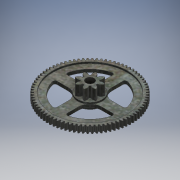
# Autodesk Inventor part: 足 初段焼結ギア　80-8
Saved by Autodesk Inventor 2016 (Build 200138000, 138)
## iProperties
Created: 2018-04-22
Part Number: 足 初段焼結ギア　80-8
Material: 鋼
Document SubType Name: Modeling
Designer: Takumi
Density: 7.85 g/cm^3
Appearance: プレート
Mass: 15.2958 g
Surface Area: 32.495 cm^2
Volume: 1.9485 cm^3
Author: Takumi
Autodesk Inventor part; units mm, degrees
(part 1 of 7)
ref_plane "YZ Plane" through (0, 0, 0) normal (1, 0, 0) x (0, 1, 0)
ref_plane "XZ Plane" through (0, 0, 0) normal (0, 1, 0) x (-1, 0, 0)
ref_plane "XY Plane" through (0, 0, 0) normal (0, 0, 1) x (1, 0, 0)
sketch "スケッチ1" plane through (0, 0, 0) normal (0, 0, 1) x (1, 0, 0)
  arc A0 (148.7771, 124.6719) -> (148.6896, 124.3741) centre (153.7892, 123.0371) ccw
  arc A1 (148.9109, 125.0429) -> (148.7771, 124.6719) centre (154.869, 122.6849) ccw
  arc A2 (149.1052, 125.4911) -> (148.9109, 125.0429) centre (155.9658, 122.2508) ccw
  arc A3 (147.2329, 124.633) -> (147.169, 124.3292) centre (152.3577, 123.3965) ccw
  arc A4 (147.3371, 125.0133) -> (147.2329, 124.633) centre (153.4618, 123.1301) ccw
  arc A5 (147.4956, 125.4754) -> (147.3371, 125.0133) centre (154.5894, 122.7834) ccw
  arc A6 (145.6964, 124.473) -> (145.6565, 124.1652) centre (150.9025, 123.6425) ccw
  arc A7 (145.7705, 124.8604) -> (145.6964, 124.473) centre (152.0241, 123.4635) ccw
  arc A8 (145.8922, 125.3335) -> (145.7705, 124.8604) centre (153.1753, 123.2064) ccw
  arc A9 (144.1772, 124.193) -> (144.1616, 123.883) centre (149.4324, 123.7735) ccw
  arc A10 (144.2207, 124.585) -> (144.1772, 124.193) centre (150.5646, 123.6831) ccw
  arc A11 (144.3049, 125.0662) -> (144.2207, 124.585) centre (151.7324, 123.517) ccw
  arc A12 (142.6846, 123.7947) -> (142.6934, 123.4844) centre (147.9566, 123.7888) ccw
  arc A13 (142.6972, 124.1889) -> (142.6846, 123.7947) centre (149.0924, 123.7875) ccw
  arc A14 (142.7435, 124.6752) -> (142.6972, 124.1889) centre (150.2696, 123.7136) ccw
  arc A15 (141.228, 123.2805) -> (141.2611, 122.9719) centre (146.4841, 123.6882) ccw
  arc A16 (141.2096, 123.6745) -> (141.228, 123.2805) centre (147.6165, 123.776) ccw
  arc A17 (141.2175, 124.1629) -> (141.2096, 123.6745) centre (148.7959, 123.7947) ccw
  arc A18 (139.8161, 122.6536) -> (139.8733, 122.3485) centre (145.024, 123.4724) ccw
  arc A19 (139.7669, 123.0449) -> (139.8161, 122.6536) centre (146.1461, 123.6488) ccw
  arc A20 (139.7365, 123.5324) -> (139.7669, 123.0449) centre (147.3204, 123.76) ccw
  arc A21 (138.4578, 121.9178) -> (138.5388, 121.6182) centre (143.5854, 123.1428) ccw
  arc A22 (138.378, 122.3041) -> (138.4578, 121.9178) centre (144.6901, 123.4067) ccw
  arc A23 (138.3095, 122.7877) -> (138.378, 122.3041) centre (145.8522, 123.6096) ccw
  arc A24 (137.1614, 121.0778) -> (137.2656, 120.7854) centre (142.1771, 122.7012) ccw
  arc A25 (137.0515, 121.4566) -> (137.1614, 121.0778) centre (143.2577, 123.051) ccw
  arc A26 (136.9453, 121.9334) -> (137.0515, 121.4566) centre (144.4002, 123.3445) ccw
  arc A27 (135.9349, 120.1386) -> (136.0617, 119.8553) centre (140.8078, 122.1506) ccw
  arc A28 (135.7957, 120.5076) -> (135.9349, 120.1386) centre (141.8576, 122.5841) ccw
  arc A29 (135.6523, 120.9746) -> (135.7957, 120.5076) centre (142.9736, 122.9663) ccw
  arc A30 (134.7859, 119.1061) -> (134.9345, 118.8336) centre (139.4859, 121.4942) ccw
  arc A31 (134.6181, 119.463) -> (134.7859, 119.1061) centre (140.4985, 122.0087) ccw
  arc A32 (134.4386, 119.9173) -> (134.6181, 119.463) centre (141.581, 122.4773) ccw
  arc A33 (133.7214, 117.9866) -> (133.891, 117.7266) centre (138.2195, 120.7361) ccw
  arc A34 (133.5261, 118.3293) -> (133.7214, 117.9866) centre (139.1886, 121.3285) ccw
  arc A35 (133.3115, 118.7681) -> (133.5261, 118.3293) centre (140.2311, 121.8806) ccw
  arc A36 (132.748, 116.7871) -> (132.9375, 116.5412) centre (137.0166, 119.881) ccw
  arc A37 (132.5265, 117.1134) -> (132.748, 116.7871) centre (137.9362, 120.5476) ccw
  arc A38 (132.2781, 117.534) -> (132.5265, 117.1134) centre (138.9321, 121.1798) ccw
  arc A39 (131.8718, 115.5148) -> (132.08, 115.2846) centre (135.8844, 118.9341) ccw
  arc A40 (131.6253, 115.8227) -> (131.8718, 115.5148) centre (136.7489, 119.6708) ccw
  arc A41 (131.3447, 116.2226) -> (131.6253, 115.8227) centre (137.6922, 120.3792) ccw
  arc A42 (131.0981, 114.1778) -> (131.3237, 113.9646) centre (134.8301, 117.9014) ccw
  arc A43 (130.8282, 114.4654) -> (131.0981, 114.1778) centre (135.6341, 118.7036) ccw
  arc A44 (130.5171, 114.842) -> (130.8282, 114.4654) centre (136.5188, 119.4838) ccw
  arc A45 (130.4316, 112.7842) -> (130.6733, 112.5893) centre (133.86, 116.7891) ccw
  arc A46 (130.14, 113.0497) -> (130.4316, 112.7842) centre (134.5986, 117.6519) ccw
  arc A47 (129.8003, 113.4007) -> (130.14, 113.0497) centre (135.4194, 118.4991) ccw
  arc A48 (129.8766, 111.3425) -> (130.1328, 111.1673) centre (132.9801, 115.6041) ccw
  arc A49 (129.5651, 111.5844) -> (129.8766, 111.3425) centre (133.6488, 116.5222) ccw
  arc A50 (129.1989, 111.9077) -> (129.5651, 111.5844) centre (134.4006, 117.4312) ccw
  arc A51 (129.4364, 109.8618) -> (129.7055, 109.7072) centre (132.196, 114.3537) ccw
  arc A52 (129.1068, 110.0785) -> (129.4364, 109.8618) centre (132.7905, 115.3215) ccw
  arc A53 (128.7164, 110.372) -> (129.1068, 110.0785) centre (133.4687, 116.2867) ccw
  arc A54 (129.1137, 108.3511) -> (129.3941, 108.2181) centre (131.5124, 113.0457) ccw
  arc A55 (128.7682, 108.5413) -> (129.1137, 108.3511) centre (132.0292, 114.0571) ccw
  arc A56 (128.3559, 108.8033) -> (128.7682, 108.5413) centre (132.6295, 115.0726) ccw
  arc A57 (128.9105, 106.8197) -> (129.2005, 106.7091) centre (130.9335, 111.6881) ccw
  arc A58 (128.5511, 106.9822) -> (128.9105, 106.8197) centre (131.3693, 112.7369) ccw
  arc A59 (128.1196, 107.2111) -> (128.5511, 106.9822) centre (131.8881, 113.7963) ccw
  arc A60 (128.8281, 105.2771) -> (129.1259, 105.1896) centre (130.4629, 110.2892) ccw
  arc A61 (128.4571, 105.4109) -> (128.8281, 105.2771) centre (130.8151, 111.369) ccw
  arc A62 (128.0089, 105.6052) -> (128.4571, 105.4109) centre (131.2492, 112.4658) ccw
  arc A63 (128.867, 103.7329) -> (129.1708, 103.669) centre (130.1035, 108.8577) ccw
  arc A64 (128.4867, 103.8371) -> (128.867, 103.7329) centre (130.3699, 109.9618) ccw
  arc A65 (128.0246, 103.9956) -> (128.4867, 103.8371) centre (130.7166, 111.0894) ccw
  arc A66 (129.027, 102.1964) -> (129.3348, 102.1565) centre (129.8575, 107.4025) ccw
  arc A67 (128.6396, 102.2705) -> (129.027, 102.1964) centre (130.0365, 108.5241) ccw
  arc A68 (128.1665, 102.3922) -> (128.6396, 102.2705) centre (130.2936, 109.6753) ccw
  arc A69 (129.307, 100.6772) -> (129.617, 100.6616) centre (129.7265, 105.9324) ccw
  arc A70 (128.915, 100.7207) -> (129.307, 100.6772) centre (129.8169, 107.0646) ccw
  arc A71 (128.4338, 100.8049) -> (128.915, 100.7207) centre (129.983, 108.2324) ccw
  arc A72 (129.7053, 99.1846) -> (130.0156, 99.1934) centre (129.7112, 104.4566) ccw
  arc A73 (129.3111, 99.1972) -> (129.7053, 99.1846) centre (129.7125, 105.5924) ccw
  arc A74 (128.8248, 99.2435) -> (129.3111, 99.1972) centre (129.7864, 106.7696) ccw
  arc A75 (130.2195, 97.728) -> (130.5281, 97.7611) centre (129.8118, 102.9841) ccw
  arc A76 (129.8255, 97.7096) -> (130.2195, 97.728) centre (129.724, 104.1165) ccw
  arc A77 (129.3371, 97.7175) -> (129.8255, 97.7096) centre (129.7053, 105.2959) ccw
  arc A78 (130.8464, 96.3161) -> (131.1515, 96.3733) centre (130.0276, 101.524) ccw
  arc A79 (130.4551, 96.2669) -> (130.8464, 96.3161) centre (129.8512, 102.6461) ccw
  arc A80 (129.9676, 96.2365) -> (130.4551, 96.2669) centre (129.74, 103.8204) ccw
  arc A81 (131.5822, 94.9578) -> (131.8818, 95.0388) centre (130.3572, 100.0854) ccw
  arc A82 (131.1959, 94.878) -> (131.5822, 94.9578) centre (130.0933, 101.1901) ccw
  arc A83 (130.7123, 94.8095) -> (131.1959, 94.878) centre (129.8904, 102.3522) ccw
  arc A84 (132.4222, 93.6614) -> (132.7146, 93.7656) centre (130.7988, 98.6771) ccw
  arc A85 (132.0434, 93.5515) -> (132.4222, 93.6614) centre (130.449, 99.7577) ccw
  arc A86 (131.5666, 93.4453) -> (132.0434, 93.5515) centre (130.1555, 100.9002) ccw
  arc A87 (133.3614, 92.4349) -> (133.6447, 92.5617) centre (131.3494, 97.3078) ccw
  arc A88 (132.9924, 92.2957) -> (133.3614, 92.4349) centre (130.9159, 98.3576) ccw
  arc A89 (132.5254, 92.1523) -> (132.9924, 92.2957) centre (130.5337, 99.4736) ccw
  arc A90 (134.3939, 91.2859) -> (134.6664, 91.4345) centre (132.0058, 95.9859) ccw
  arc A91 (134.037, 91.1181) -> (134.3939, 91.2859) centre (131.4913, 96.9985) ccw
  arc A92 (133.5827, 90.9386) -> (134.037, 91.1181) centre (131.0227, 98.081) ccw
  arc A93 (135.5134, 90.2214) -> (135.7734, 90.391) centre (132.7639, 94.7195) ccw
  arc A94 (135.1707, 90.0261) -> (135.5134, 90.2214) centre (132.1715, 95.6886) ccw
  arc A95 (134.7319, 89.8115) -> (135.1707, 90.0261) centre (131.6194, 96.7311) ccw
  arc A96 (136.7129, 89.248) -> (136.9588, 89.4375) centre (133.619, 93.5166) ccw
  arc A97 (136.3866, 89.0265) -> (136.7129, 89.248) centre (132.9524, 94.4362) ccw
  arc A98 (135.966, 88.7781) -> (136.3866, 89.0265) centre (132.3202, 95.4321) ccw
  arc A99 (137.9852, 88.3718) -> (138.2154, 88.58) centre (134.5659, 92.3844) ccw
  arc A100 (137.6773, 88.1253) -> (137.9852, 88.3718) centre (133.8292, 93.2489) ccw
  arc A101 (137.2774, 87.8447) -> (137.6773, 88.1253) centre (133.1208, 94.1922) ccw
  arc A102 (139.3222, 87.5981) -> (139.5354, 87.8237) centre (135.5986, 91.3301) ccw
  arc A103 (139.0346, 87.3282) -> (139.3222, 87.5981) centre (134.7964, 92.1341) ccw
  arc A104 (138.658, 87.0171) -> (139.0346, 87.3282) centre (134.0162, 93.0188) ccw
  arc A105 (140.7158, 86.9316) -> (140.9107, 87.1733) centre (136.7109, 90.36) ccw
  arc A106 (140.4503, 86.64) -> (140.7158, 86.9316) centre (135.8481, 91.0986) ccw
  arc A107 (140.0993, 86.3003) -> (140.4503, 86.64) centre (135.0009, 91.9194) ccw
  arc A108 (142.1575, 86.3766) -> (142.3327, 86.6328) centre (137.8959, 89.4801) ccw
  arc A109 (141.9156, 86.0651) -> (142.1575, 86.3766) centre (136.9778, 90.1488) ccw
  arc A110 (141.5923, 85.6989) -> (141.9156, 86.0651) centre (136.0688, 90.9006) ccw
  arc A111 (143.6382, 85.9364) -> (143.7928, 86.2055) centre (139.1463, 88.696) ccw
  arc A112 (143.4215, 85.6068) -> (143.6382, 85.9364) centre (138.1785, 89.2905) ccw
  arc A113 (143.128, 85.2164) -> (143.4215, 85.6068) centre (137.2133, 89.9687) ccw
  arc A114 (145.1489, 85.6137) -> (145.2819, 85.8941) centre (140.4543, 88.0124) ccw
  arc A115 (144.9587, 85.2682) -> (145.1489, 85.6137) centre (139.4429, 88.5292) ccw
  arc A116 (144.6967, 84.8559) -> (144.9587, 85.2682) centre (138.4274, 89.1295) ccw
  arc A117 (146.6803, 85.4105) -> (146.7909, 85.7005) centre (141.8119, 87.4335) ccw
  arc A118 (146.5178, 85.0511) -> (146.6803, 85.4105) centre (140.7631, 87.8693) ccw
  arc A119 (146.2889, 84.6196) -> (146.5178, 85.0511) centre (139.7037, 88.3881) ccw
  arc A120 (148.2229, 85.3281) -> (148.3104, 85.6259) centre (143.2108, 86.9629) ccw
  arc A121 (148.0891, 84.9571) -> (148.2229, 85.3281) centre (142.131, 87.3151) ccw
  arc A122 (147.8948, 84.5089) -> (148.0891, 84.9571) centre (141.0342, 87.7492) ccw
  arc A123 (149.7671, 85.367) -> (149.831, 85.6708) centre (144.6423, 86.6035) ccw
  arc A124 (149.6629, 84.9867) -> (149.7671, 85.367) centre (143.5382, 86.8699) ccw
  arc A125 (149.5044, 84.5246) -> (149.6629, 84.9867) centre (142.4106, 87.2166) ccw
  arc A126 (151.3036, 85.527) -> (151.3435, 85.8348) centre (146.0975, 86.3575) ccw
  arc A127 (151.2295, 85.1396) -> (151.3036, 85.527) centre (144.9759, 86.5365) ccw
  arc A128 (151.1078, 84.6665) -> (151.2295, 85.1396) centre (143.8247, 86.7936) ccw
  arc A129 (152.8228, 85.807) -> (152.8384, 86.117) centre (147.5676, 86.2265) ccw
  arc A130 (152.7793, 85.415) -> (152.8228, 85.807) centre (146.4354, 86.3169) ccw
  arc A131 (152.6951, 84.9338) -> (152.7793, 85.415) centre (145.2676, 86.483) ccw
  arc A132 (154.3154, 86.2053) -> (154.3066, 86.5156) centre (149.0434, 86.2112) ccw
  arc A133 (154.3028, 85.8111) -> (154.3154, 86.2053) centre (147.9076, 86.2125) ccw
  arc A134 (154.2565, 85.3248) -> (154.3028, 85.8111) centre (146.7304, 86.2864) ccw
  arc A135 (155.772, 86.7195) -> (155.7389, 87.0281) centre (150.5159, 86.3118) ccw
  arc A136 (155.7904, 86.3255) -> (155.772, 86.7195) centre (149.3835, 86.224) ccw
  arc A137 (155.7825, 85.8371) -> (155.7904, 86.3255) centre (148.2041, 86.2053) ccw
  arc A138 (157.1839, 87.3464) -> (157.1267, 87.6515) centre (151.976, 86.5276) ccw
  arc A139 (157.2331, 86.9551) -> (157.1839, 87.3464) centre (150.8539, 86.3512) ccw
  arc A140 (157.2635, 86.4676) -> (157.2331, 86.9551) centre (149.6796, 86.24) ccw
  arc A141 (158.5422, 88.0822) -> (158.4612, 88.3818) centre (153.4146, 86.8572) ccw
  arc A142 (158.622, 87.6959) -> (158.5422, 88.0822) centre (152.3099, 86.5933) ccw
  arc A143 (158.6905, 87.2123) -> (158.622, 87.6959) centre (151.1478, 86.3904) ccw
  arc A144 (159.8386, 88.9222) -> (159.7344, 89.2146) centre (154.8229, 87.2988) ccw
  arc A145 (159.9485, 88.5434) -> (159.8386, 88.9222) centre (153.7423, 86.949) ccw
  arc A146 (160.0547, 88.0666) -> (159.9485, 88.5434) centre (152.5998, 86.6555) ccw
  arc A147 (161.0651, 89.8614) -> (160.9383, 90.1447) centre (156.1922, 87.8494) ccw
  arc A148 (161.2043, 89.4924) -> (161.0651, 89.8614) centre (155.1424, 87.4159) ccw
  arc A149 (161.3477, 89.0254) -> (161.2043, 89.4924) centre (154.0264, 87.0337) ccw
  arc A150 (162.2141, 90.8939) -> (162.0655, 91.1664) centre (157.5141, 88.5058) ccw
  arc A151 (162.3819, 90.537) -> (162.2141, 90.8939) centre (156.5015, 87.9913) ccw
  arc A152 (162.5614, 90.0827) -> (162.3819, 90.537) centre (155.419, 87.5227) ccw
  arc A153 (163.2786, 92.0134) -> (163.109, 92.2734) centre (158.7805, 89.2639) ccw
  arc A154 (163.4738, 91.6707) -> (163.2786, 92.0134) centre (157.8114, 88.6715) ccw
  arc A155 (163.6885, 91.2319) -> (163.4738, 91.6707) centre (156.7689, 88.1194) ccw
  arc A156 (164.252, 93.2129) -> (164.0625, 93.4588) centre (159.9834, 90.119) ccw
  arc A157 (164.4735, 92.8866) -> (164.252, 93.2129) centre (159.0638, 89.4524) ccw
  arc A158 (164.7219, 92.466) -> (164.4735, 92.8866) centre (158.0679, 88.8202) ccw
  arc A159 (165.1282, 94.4852) -> (164.92, 94.7154) centre (161.1156, 91.0659) ccw
  arc A160 (165.3747, 94.1773) -> (165.1282, 94.4852) centre (160.2511, 90.3292) ccw
  arc A161 (165.6553, 93.7774) -> (165.3747, 94.1773) centre (159.3078, 89.6208) ccw
  arc A162 (165.9019, 95.8222) -> (165.6763, 96.0354) centre (162.1699, 92.0986) ccw
  arc A163 (166.1718, 95.5346) -> (165.9019, 95.8222) centre (161.3659, 91.2964) ccw
  arc A164 (166.4829, 95.158) -> (166.1718, 95.5346) centre (160.4812, 90.5162) ccw
  arc A165 (166.5684, 97.2158) -> (166.3267, 97.4107) centre (163.14, 93.2109) ccw
  arc A166 (166.86, 96.9503) -> (166.5684, 97.2158) centre (162.4014, 92.3481) ccw
  arc A167 (167.1997, 96.5993) -> (166.86, 96.9503) centre (161.5806, 91.5009) ccw
  arc A168 (167.1234, 98.6575) -> (166.8672, 98.8327) centre (164.0199, 94.3959) ccw
  arc A169 (167.4349, 98.4156) -> (167.1234, 98.6575) centre (163.3512, 93.4778) ccw
  arc A170 (167.8011, 98.0923) -> (167.4349, 98.4156) centre (162.5994, 92.5688) ccw
  arc A171 (167.5636, 100.1382) -> (167.2945, 100.2928) centre (164.804, 95.6463) ccw
  arc A172 (167.8932, 99.9215) -> (167.5636, 100.1382) centre (164.2095, 94.6785) ccw
  arc A173 (168.2836, 99.628) -> (167.8932, 99.9215) centre (163.5313, 93.7133) ccw
  arc A174 (167.8863, 101.6489) -> (167.6059, 101.7819) centre (165.4876, 96.9543) ccw
  arc A175 (168.2318, 101.4587) -> (167.8863, 101.6489) centre (164.9708, 95.9429) ccw
  arc A176 (168.6441, 101.1967) -> (168.2318, 101.4587) centre (164.3705, 94.9274) ccw
  arc A177 (168.0895, 103.1803) -> (167.7995, 103.2909) centre (166.0665, 98.3119) ccw
  arc A178 (168.4489, 103.0178) -> (168.0895, 103.1803) centre (165.6307, 97.2631) ccw
  arc A179 (168.8804, 102.7889) -> (168.4489, 103.0178) centre (165.1119, 96.2037) ccw
  arc A180 (168.1719, 104.7229) -> (167.8741, 104.8104) centre (166.5371, 99.7108) ccw
  arc A181 (168.5429, 104.5891) -> (168.1719, 104.7229) centre (166.1849, 98.631) ccw
  arc A182 (168.9911, 104.3948) -> (168.5429, 104.5891) centre (165.7508, 97.5342) ccw
  arc A183 (168.133, 106.2671) -> (167.8292, 106.331) centre (166.8965, 101.1423) ccw
  arc A184 (168.5133, 106.1629) -> (168.133, 106.2671) centre (166.6301, 100.0382) ccw
  arc A185 (168.9754, 106.0044) -> (168.5133, 106.1629) centre (166.2834, 98.9106) ccw
  arc A186 (167.973, 107.8036) -> (167.6652, 107.8435) centre (167.1425, 102.5975) ccw
  arc A187 (168.3604, 107.7295) -> (167.973, 107.8036) centre (166.9635, 101.4759) ccw
  arc A188 (168.8335, 107.6078) -> (168.3604, 107.7295) centre (166.7064, 100.3247) ccw
  arc A189 (167.693, 109.3228) -> (167.383, 109.3384) centre (167.2735, 104.0676) ccw
  arc A190 (168.085, 109.2793) -> (167.693, 109.3228) centre (167.1831, 102.9354) ccw
  arc A191 (168.5662, 109.1951) -> (168.085, 109.2793) centre (167.017, 101.7676) ccw
  arc A192 (167.2947, 110.8154) -> (166.9844, 110.8066) centre (167.2888, 105.5434) ccw
  arc A193 (167.6889, 110.8028) -> (167.2947, 110.8154) centre (167.2875, 104.4076) ccw
  arc A194 (168.1752, 110.7565) -> (167.6889, 110.8028) centre (167.2136, 103.2304) ccw
  arc A195 (166.7805, 112.272) -> (166.4719, 112.2389) centre (167.1882, 107.0159) ccw
  arc A196 (167.1745, 112.2904) -> (166.7805, 112.272) centre (167.276, 105.8835) ccw
  arc A197 (167.6629, 112.2825) -> (167.1745, 112.2904) centre (167.2947, 104.7041) ccw
  arc A198 (166.1536, 113.6839) -> (165.8485, 113.6267) centre (166.9724, 108.476) ccw
  arc A199 (166.5449, 113.7331) -> (166.1536, 113.6839) centre (167.1488, 107.3539) ccw
  arc A200 (167.0324, 113.7635) -> (166.5449, 113.7331) centre (167.26, 106.1796) ccw
  arc A201 (165.4178, 115.0422) -> (165.1182, 114.9612) centre (166.6428, 109.9146) ccw
  arc A202 (165.8041, 115.122) -> (165.4178, 115.0422) centre (166.9067, 108.8099) ccw
  arc A203 (166.2877, 115.1905) -> (165.8041, 115.122) centre (167.1096, 107.6478) ccw
  arc A204 (164.5778, 116.3386) -> (164.2854, 116.2344) centre (166.2012, 111.3229) ccw
  arc A205 (164.9566, 116.4485) -> (164.5778, 116.3386) centre (166.551, 110.2423) ccw
  arc A206 (165.4334, 116.5547) -> (164.9566, 116.4485) centre (166.8445, 109.0998) ccw
  arc A207 (163.6386, 117.5651) -> (163.3553, 117.4383) centre (165.6506, 112.6922) ccw
  arc A208 (164.0076, 117.7043) -> (163.6386, 117.5651) centre (166.0841, 111.6424) ccw
  arc A209 (164.4746, 117.8477) -> (164.0076, 117.7043) centre (166.4663, 110.5264) ccw
  arc A210 (162.6061, 118.7141) -> (162.3336, 118.5655) centre (164.9942, 114.0141) ccw
  arc A211 (162.963, 118.8819) -> (162.6061, 118.7141) centre (165.5087, 113.0015) ccw
  arc A212 (163.4173, 119.0614) -> (162.963, 118.8819) centre (165.9773, 111.919) ccw
  arc A213 (161.4866, 119.7786) -> (161.2266, 119.609) centre (164.2361, 115.2805) ccw
  arc A214 (161.8293, 119.9739) -> (161.4866, 119.7786) centre (164.8285, 114.3114) ccw
  arc A215 (162.2681, 120.1885) -> (161.8293, 119.9739) centre (165.3806, 113.2689) ccw
  arc A216 (160.2871, 120.752) -> (160.0412, 120.5625) centre (163.381, 116.4834) ccw
  arc A217 (160.6134, 120.9735) -> (160.2871, 120.752) centre (164.0476, 115.5638) ccw
  arc A218 (161.034, 121.2219) -> (160.6134, 120.9735) centre (164.6798, 114.5679) ccw
  arc A219 (159.0148, 121.6282) -> (158.7846, 121.42) centre (162.4341, 117.6156) ccw
  arc A220 (159.3227, 121.8747) -> (159.0148, 121.6282) centre (163.1708, 116.7511) ccw
  arc A221 (159.7226, 122.1553) -> (159.3227, 121.8747) centre (163.8792, 115.8078) ccw
  arc A222 (157.6778, 122.4019) -> (157.4646, 122.1763) centre (161.4014, 118.6699) ccw
  arc A223 (157.9654, 122.6718) -> (157.6778, 122.4019) centre (162.2036, 117.8659) ccw
  arc A224 (158.342, 122.9829) -> (157.9654, 122.6718) centre (162.9838, 116.9812) ccw
  arc A225 (156.2842, 123.0684) -> (156.0893, 122.8267) centre (160.2891, 119.64) ccw
  arc A226 (156.5497, 123.36) -> (156.2842, 123.0684) centre (161.1519, 118.9014) ccw
  arc A227 (156.9007, 123.6997) -> (156.5497, 123.36) centre (161.9991, 118.0806) ccw
  arc A228 (154.8425, 123.6234) -> (154.6673, 123.3672) centre (159.1041, 120.5199) ccw
  arc A229 (155.0844, 123.9349) -> (154.8425, 123.6234) centre (160.0222, 119.8512) ccw
  arc A230 (155.4077, 124.3011) -> (155.0844, 123.9349) centre (160.9312, 119.0994) ccw
  arc A231 (153.3618, 124.0636) -> (153.2072, 123.7945) centre (157.8537, 121.304) ccw
  arc A232 (153.5785, 124.3932) -> (153.3618, 124.0636) centre (158.8215, 120.7095) ccw
  arc A233 (153.872, 124.7836) -> (153.5785, 124.3932) centre (159.7867, 120.0313) ccw
  arc A234 (151.8511, 124.3863) -> (151.7181, 124.1059) centre (156.5457, 121.9876) ccw
  arc A235 (152.0413, 124.7318) -> (151.8511, 124.3863) centre (157.5571, 121.4708) ccw
  arc A236 (152.3033, 125.1441) -> (152.0413, 124.7318) centre (158.5726, 120.8705) ccw
  arc A237 (150.3197, 124.5895) -> (150.2091, 124.2995) centre (155.1881, 122.5665) ccw
  arc A238 (150.4822, 124.9489) -> (150.3197, 124.5895) centre (156.2369, 122.1307) ccw
  arc A239 (150.7111, 125.3804) -> (150.4822, 124.9489) centre (157.2963, 121.6119) ccw
  arc A240 (148.3104, 124.3741) -> (148.2229, 124.6719) centre (143.2108, 123.0371) ccw
  arc A241 (148.2229, 124.6719) -> (148.0891, 125.0429) centre (142.131, 122.6849) ccw
  arc A242 (148.0891, 125.0429) -> (147.8948, 125.4911) centre (141.0342, 122.2508) ccw
  arc A243 (146.7909, 124.2995) -> (146.6803, 124.5895) centre (141.8119, 122.5665) ccw
  arc A244 (146.6803, 124.5895) -> (146.5178, 124.9489) centre (140.7631, 122.1307) ccw
  arc A245 (146.5178, 124.9489) -> (146.2889, 125.3804) centre (139.7037, 121.6119) ccw
  arc A246 (145.2819, 124.1059) -> (145.1489, 124.3863) centre (140.4543, 121.9876) ccw
  arc A247 (145.1489, 124.3863) -> (144.9587, 124.7318) centre (139.4429, 121.4708) ccw
  arc A248 (144.9587, 124.7318) -> (144.6967, 125.1441) centre (138.4274, 120.8705) ccw
  arc A249 (143.7928, 123.7945) -> (143.6382, 124.0636) centre (139.1463, 121.304) ccw
  arc A250 (143.6382, 124.0636) -> (143.4215, 124.3932) centre (138.1785, 120.7095) ccw
  arc A251 (143.4215, 124.3932) -> (143.128, 124.7836) centre (137.2133, 120.0313) ccw
  arc A252 (142.3327, 123.3672) -> (142.1575, 123.6234) centre (137.8959, 120.5199) ccw
  arc A253 (142.1575, 123.6234) -> (141.9156, 123.9349) centre (136.9778, 119.8512) ccw
  arc A254 (141.9156, 123.9349) -> (141.5923, 124.3011) centre (136.0688, 119.0994) ccw
  arc A255 (140.9107, 122.8267) -> (140.7158, 123.0684) centre (136.7109, 119.64) ccw
  arc A256 (140.7158, 123.0684) -> (140.4503, 123.36) centre (135.8481, 118.9014) ccw
  arc A257 (140.4503, 123.36) -> (140.0993, 123.6997) centre (135.0009, 118.0806) ccw
  arc A258 (139.5354, 122.1763) -> (139.3222, 122.4019) centre (135.5986, 118.6699) ccw
  arc A259 (139.3222, 122.4019) -> (139.0346, 122.6718) centre (134.7964, 117.8659) ccw
  arc A260 (139.0346, 122.6718) -> (138.658, 122.9829) centre (134.0162, 116.9812) ccw
  arc A261 (138.2154, 121.42) -> (137.9852, 121.6282) centre (134.5659, 117.6156) ccw
  arc A262 (137.9852, 121.6282) -> (137.6773, 121.8747) centre (133.8292, 116.7511) ccw
  arc A263 (137.6773, 121.8747) -> (137.2774, 122.1553) centre (133.1208, 115.8078) ccw
  arc A264 (136.9588, 120.5625) -> (136.7129, 120.752) centre (133.619, 116.4834) ccw
  arc A265 (136.7129, 120.752) -> (136.3866, 120.9735) centre (132.9524, 115.5638) ccw
  arc A266 (136.3866, 120.9735) -> (135.966, 121.2219) centre (132.3202, 114.5679) ccw
  arc A267 (135.7734, 119.609) -> (135.5134, 119.7786) centre (132.7639, 115.2805) ccw
  arc A268 (135.5134, 119.7786) -> (135.1707, 119.9739) centre (132.1715, 114.3114) ccw
  arc A269 (135.1707, 119.9739) -> (134.7319, 120.1885) centre (131.6194, 113.2689) ccw
  arc A270 (134.6664, 118.5655) -> (134.3939, 118.7141) centre (132.0058, 114.0141) ccw
  arc A271 (134.3939, 118.7141) -> (134.037, 118.8819) centre (131.4913, 113.0015) ccw
  arc A272 (134.037, 118.8819) -> (133.5827, 119.0614) centre (131.0227, 111.919) ccw
  arc A273 (133.6447, 117.4383) -> (133.3614, 117.5651) centre (131.3494, 112.6922) ccw
  arc A274 (133.3614, 117.5651) -> (132.9924, 117.7043) centre (130.9159, 111.6424) ccw
  arc A275 (132.9924, 117.7043) -> (132.5254, 117.8477) centre (130.5337, 110.5264) ccw
  arc A276 (132.7146, 116.2344) -> (132.4222, 116.3386) centre (130.7988, 111.3229) ccw
  arc A277 (132.4222, 116.3386) -> (132.0434, 116.4485) centre (130.449, 110.2423) ccw
  arc A278 (132.0434, 116.4485) -> (131.5666, 116.5547) centre (130.1555, 109.0998) ccw
  arc A279 (131.8818, 114.9612) -> (131.5822, 115.0422) centre (130.3572, 109.9146) ccw
  arc A280 (131.5822, 115.0422) -> (131.1959, 115.122) centre (130.0933, 108.8099) ccw
  arc A281 (131.1959, 115.122) -> (130.7123, 115.1905) centre (129.8904, 107.6478) ccw
  arc A282 (131.1515, 113.6267) -> (130.8464, 113.6839) centre (130.0276, 108.476) ccw
  arc A283 (130.8464, 113.6839) -> (130.4551, 113.7331) centre (129.8512, 107.3539) ccw
  arc A284 (130.4551, 113.7331) -> (129.9676, 113.7635) centre (129.74, 106.1796) ccw
  arc A285 (130.5281, 112.2389) -> (130.2195, 112.272) centre (129.8118, 107.0159) ccw
  arc A286 (130.2195, 112.272) -> (129.8255, 112.2904) centre (129.724, 105.8835) ccw
  arc A287 (129.8255, 112.2904) -> (129.3371, 112.2825) centre (129.7053, 104.7041) ccw
  arc A288 (130.0156, 110.8066) -> (129.7053, 110.8154) centre (129.7112, 105.5434) ccw
  arc A289 (129.7053, 110.8154) -> (129.3111, 110.8028) centre (129.7125, 104.4076) ccw
  arc A290 (129.3111, 110.8028) -> (128.8248, 110.7565) centre (129.7864, 103.2304) ccw
  arc A291 (129.617, 109.3384) -> (129.307, 109.3228) centre (129.7265, 104.0676) ccw
  arc A292 (129.307, 109.3228) -> (128.915, 109.2793) centre (129.8169, 102.9354) ccw
  arc A293 (128.915, 109.2793) -> (128.4338, 109.1951) centre (129.983, 101.7676) ccw
  arc A294 (129.3348, 107.8435) -> (129.027, 107.8036) centre (129.8575, 102.5975) ccw
  arc A295 (129.027, 107.8036) -> (128.6396, 107.7295) centre (130.0365, 101.4759) ccw
  arc A296 (128.6396, 107.7295) -> (128.1665, 107.6078) centre (130.2936, 100.3247) ccw
  arc A297 (129.1708, 106.331) -> (128.867, 106.2671) centre (130.1035, 101.1423) ccw
  arc A298 (128.867, 106.2671) -> (128.4867, 106.1629) centre (130.3699, 100.0382) ccw
  arc A299 (128.4867, 106.1629) -> (128.0246, 106.0044) centre (130.7166, 98.9106) ccw
  arc A300 (129.1259, 104.8104) -> (128.8281, 104.7229) centre (130.4629, 99.7108) ccw
  arc A301 (128.8281, 104.7229) -> (128.4571, 104.5891) centre (130.8151, 98.631) ccw
  arc A302 (128.4571, 104.5891) -> (128.0089, 104.3948) centre (131.2492, 97.5342) ccw
  arc A303 (129.2005, 103.2909) -> (128.9105, 103.1803) centre (130.9335, 98.3119) ccw
  arc A304 (128.9105, 103.1803) -> (128.5511, 103.0178) centre (131.3693, 97.2631) ccw
  arc A305 (128.5511, 103.0178) -> (128.1196, 102.7889) centre (131.8881, 96.2037) ccw
  arc A306 (129.3941, 101.7819) -> (129.1137, 101.6489) centre (131.5124, 96.9543) ccw
  arc A307 (129.1137, 101.6489) -> (128.7682, 101.4587) centre (132.0292, 95.9429) ccw
  arc A308 (128.7682, 101.4587) -> (128.3559, 101.1967) centre (132.6295, 94.9274) ccw
  arc A309 (129.7055, 100.2928) -> (129.4364, 100.1382) centre (132.196, 95.6463) ccw
  arc A310 (129.4364, 100.1382) -> (129.1068, 99.9215) centre (132.7905, 94.6785) ccw
  arc A311 (129.1068, 99.9215) -> (128.7164, 99.628) centre (133.4687, 93.7133) ccw
  arc A312 (130.1328, 98.8327) -> (129.8766, 98.6575) centre (132.9801, 94.3959) ccw
  arc A313 (129.8766, 98.6575) -> (129.5651, 98.4156) centre (133.6488, 93.4778) ccw
  arc A314 (129.5651, 98.4156) -> (129.1989, 98.0923) centre (134.4006, 92.5688) ccw
  arc A315 (130.6733, 97.4107) -> (130.4316, 97.2158) centre (133.86, 93.2109) ccw
  arc A316 (130.4316, 97.2158) -> (130.14, 96.9503) centre (134.5986, 92.3481) ccw
  arc A317 (130.14, 96.9503) -> (129.8003, 96.5993) centre (135.4194, 91.5009) ccw
  arc A318 (131.3237, 96.0354) -> (131.0981, 95.8222) centre (134.8301, 92.0986) ccw
  arc A319 (131.0981, 95.8222) -> (130.8282, 95.5346) centre (135.6341, 91.2964) ccw
  arc A320 (130.8282, 95.5346) -> (130.5171, 95.158) centre (136.5188, 90.5162) ccw
  arc A321 (132.08, 94.7154) -> (131.8718, 94.4852) centre (135.8844, 91.0659) ccw
  arc A322 (131.8718, 94.4852) -> (131.6253, 94.1773) centre (136.7489, 90.3292) ccw
  arc A323 (131.6253, 94.1773) -> (131.3447, 93.7774) centre (137.6922, 89.6208) ccw
  arc A324 (132.9375, 93.4588) -> (132.748, 93.2129) centre (137.0166, 90.119) ccw
  arc A325 (132.748, 93.2129) -> (132.5265, 92.8866) centre (137.9362, 89.4524) ccw
  arc A326 (132.5265, 92.8866) -> (132.2781, 92.466) centre (138.9321, 88.8202) ccw
  arc A327 (133.891, 92.2734) -> (133.7214, 92.0134) centre (138.2195, 89.2639) ccw
  arc A328 (133.7214, 92.0134) -> (133.5261, 91.6707) centre (139.1886, 88.6715) ccw
  arc A329 (133.5261, 91.6707) -> (133.3115, 91.2319) centre (140.2311, 88.1194) ccw
  arc A330 (134.9345, 91.1664) -> (134.7859, 90.8939) centre (139.4859, 88.5058) ccw
  arc A331 (134.7859, 90.8939) -> (134.6181, 90.537) centre (140.4985, 87.9913) ccw
  arc A332 (134.6181, 90.537) -> (134.4386, 90.0827) centre (141.581, 87.5227) ccw
  arc A333 (136.0617, 90.1447) -> (135.9349, 89.8614) centre (140.8078, 87.8494) ccw
  arc A334 (135.9349, 89.8614) -> (135.7957, 89.4924) centre (141.8576, 87.4159) ccw
  arc A335 (135.7957, 89.4924) -> (135.6523, 89.0254) centre (142.9736, 87.0337) ccw
  arc A336 (137.2656, 89.2146) -> (137.1614, 88.9222) centre (142.1771, 87.2988) ccw
  arc A337 (137.1614, 88.9222) -> (137.0515, 88.5434) centre (143.2577, 86.949) ccw
  arc A338 (137.0515, 88.5434) -> (136.9453, 88.0666) centre (144.4002, 86.6555) ccw
  arc A339 (138.5388, 88.3818) -> (138.4578, 88.0822) centre (143.5854, 86.8572) ccw
  arc A340 (138.4578, 88.0822) -> (138.378, 87.6959) centre (144.6901, 86.5933) ccw
  arc A341 (138.378, 87.6959) -> (138.3095, 87.2123) centre (145.8522, 86.3904) ccw
  arc A342 (139.8733, 87.6515) -> (139.8161, 87.3464) centre (145.024, 86.5276) ccw
  arc A343 (139.8161, 87.3464) -> (139.7669, 86.9551) centre (146.1461, 86.3512) ccw
  arc A344 (139.7669, 86.9551) -> (139.7365, 86.4676) centre (147.3204, 86.24) ccw
  arc A345 (141.2611, 87.0281) -> (141.228, 86.7195) centre (146.4841, 86.3118) ccw
  arc A346 (141.228, 86.7195) -> (141.2096, 86.3255) centre (147.6165, 86.224) ccw
  arc A347 (141.2096, 86.3255) -> (141.2175, 85.8371) centre (148.7959, 86.2053) ccw
  arc A348 (142.6934, 86.5156) -> (142.6846, 86.2053) centre (147.9566, 86.2112) ccw
  arc A349 (142.6846, 86.2053) -> (142.6972, 85.8111) centre (149.0924, 86.2125) ccw
  arc A350 (142.6972, 85.8111) -> (142.7435, 85.3248) centre (150.2696, 86.2864) ccw
  arc A351 (144.1616, 86.117) -> (144.1772, 85.807) centre (149.4324, 86.2265) ccw
  arc A352 (144.1772, 85.807) -> (144.2207, 85.415) centre (150.5646, 86.3169) ccw
  arc A353 (144.2207, 85.415) -> (144.3049, 84.9338) centre (151.7324, 86.483) ccw
  arc A354 (145.6565, 85.8348) -> (145.6964, 85.527) centre (150.9025, 86.3575) ccw
  arc A355 (145.6964, 85.527) -> (145.7705, 85.1396) centre (152.0241, 86.5365) ccw
  arc A356 (145.7705, 85.1396) -> (145.8922, 84.6665) centre (153.1753, 86.7936) ccw
  arc A357 (147.169, 85.6708) -> (147.2329, 85.367) centre (152.3577, 86.6035) ccw
  arc A358 (147.2329, 85.367) -> (147.3371, 84.9867) centre (153.4618, 86.8699) ccw
  arc A359 (147.3371, 84.9867) -> (147.4956, 84.5246) centre (154.5894, 87.2166) ccw
  arc A360 (148.6896, 85.6259) -> (148.7771, 85.3281) centre (153.7892, 86.9629) ccw
  arc A361 (148.7771, 85.3281) -> (148.9109, 84.9571) centre (154.869, 87.3151) ccw
  arc A362 (148.9109, 84.9571) -> (149.1052, 84.5089) centre (155.9658, 87.7492) ccw
  arc A363 (150.2091, 85.7005) -> (150.3197, 85.4105) centre (155.1881, 87.4335) ccw
  arc A364 (150.3197, 85.4105) -> (150.4822, 85.0511) centre (156.2369, 87.8693) ccw
  arc A365 (150.4822, 85.0511) -> (150.7111, 84.6196) centre (157.2963, 88.3881) ccw
  arc A366 (151.7181, 85.8941) -> (151.8511, 85.6137) centre (156.5457, 88.0124) ccw
  arc A367 (151.8511, 85.6137) -> (152.0413, 85.2682) centre (157.5571, 88.5292) ccw
  arc A368 (152.0413, 85.2682) -> (152.3033, 84.8559) centre (158.5726, 89.1295) ccw
  arc A369 (153.2072, 86.2055) -> (153.3618, 85.9364) centre (157.8537, 88.696) ccw
  arc A370 (153.3618, 85.9364) -> (153.5785, 85.6068) centre (158.8215, 89.2905) ccw
  arc A371 (153.5785, 85.6068) -> (153.872, 85.2164) centre (159.7867, 89.9687) ccw
  arc A372 (154.6673, 86.6328) -> (154.8425, 86.3766) centre (159.1041, 89.4801) ccw
  arc A373 (154.8425, 86.3766) -> (155.0844, 86.0651) centre (160.0222, 90.1488) ccw
  arc A374 (155.0844, 86.0651) -> (155.4077, 85.6989) centre (160.9312, 90.9006) ccw
  arc A375 (156.0893, 87.1733) -> (156.2842, 86.9316) centre (160.2891, 90.36) ccw
  arc A376 (156.2842, 86.9316) -> (156.5497, 86.64) centre (161.1519, 91.0986) ccw
  arc A377 (156.5497, 86.64) -> (156.9007, 86.3003) centre (161.9991, 91.9194) ccw
  arc A378 (157.4646, 87.8237) -> (157.6778, 87.5981) centre (161.4014, 91.3301) ccw
  arc A379 (157.6778, 87.5981) -> (157.9654, 87.3282) centre (162.2036, 92.1341) ccw
  arc A380 (157.9654, 87.3282) -> (158.342, 87.0171) centre (162.9838, 93.0188) ccw
  arc A381 (158.7846, 88.58) -> (159.0148, 88.3718) centre (162.4341, 92.3844) ccw
  arc A382 (159.0148, 88.3718) -> (159.3227, 88.1253) centre (163.1708, 93.2489) ccw
  arc A383 (159.3227, 88.1253) -> (159.7226, 87.8447) centre (163.8792, 94.1922) ccw
  arc A384 (160.0412, 89.4375) -> (160.2871, 89.248) centre (163.381, 93.5166) ccw
  arc A385 (160.2871, 89.248) -> (160.6134, 89.0265) centre (164.0476, 94.4362) ccw
  arc A386 (160.6134, 89.0265) -> (161.034, 88.7781) centre (164.6798, 95.4321) ccw
  arc A387 (161.2266, 90.391) -> (161.4866, 90.2214) centre (164.2361, 94.7195) ccw
  arc A388 (161.4866, 90.2214) -> (161.8293, 90.0261) centre (164.8285, 95.6886) ccw
  arc A389 (161.8293, 90.0261) -> (162.2681, 89.8115) centre (165.3806, 96.7311) ccw
  arc A390 (162.3336, 91.4345) -> (162.6061, 91.2859) centre (164.9942, 95.9859) ccw
  arc A391 (162.6061, 91.2859) -> (162.963, 91.1181) centre (165.5087, 96.9985) ccw
  arc A392 (162.963, 91.1181) -> (163.4173, 90.9386) centre (165.9773, 98.081) ccw
  arc A393 (163.3553, 92.5617) -> (163.6386, 92.4349) centre (165.6506, 97.3078) ccw
  arc A394 (163.6386, 92.4349) -> (164.0076, 92.2957) centre (166.0841, 98.3576) ccw
  arc A395 (164.0076, 92.2957) -> (164.4746, 92.1523) centre (166.4663, 99.4736) ccw
  arc A396 (164.2854, 93.7656) -> (164.5778, 93.6614) centre (166.2012, 98.6771) ccw
  arc A397 (164.5778, 93.6614) -> (164.9566, 93.5515) centre (166.551, 99.7577) ccw
  arc A398 (164.9566, 93.5515) -> (165.4334, 93.4453) centre (166.8445, 100.9002) ccw
  arc A399 (165.1182, 95.0388) -> (165.4178, 94.9578) centre (166.6428, 100.0854) ccw
  arc A400 (165.4178, 94.9578) -> (165.8041, 94.878) centre (166.9067, 101.1901) ccw
  arc A401 (165.8041, 94.878) -> (166.2877, 94.8095) centre (167.1096, 102.3522) ccw
  arc A402 (165.8485, 96.3733) -> (166.1536, 96.3161) centre (166.9724, 101.524) ccw
  arc A403 (166.1536, 96.3161) -> (166.5449, 96.2669) centre (167.1488, 102.6461) ccw
  arc A404 (166.5449, 96.2669) -> (167.0324, 96.2365) centre (167.26, 103.8204) ccw
  arc A405 (166.4719, 97.7611) -> (166.7805, 97.728) centre (167.1882, 102.9841) ccw
  arc A406 (166.7805, 97.728) -> (167.1745, 97.7096) centre (167.276, 104.1165) ccw
  arc A407 (167.1745, 97.7096) -> (167.6629, 97.7175) centre (167.2947, 105.2959) ccw
  arc A408 (166.9844, 99.1934) -> (167.2947, 99.1846) centre (167.2888, 104.4566) ccw
  arc A409 (167.2947, 99.1846) -> (167.6889, 99.1972) centre (167.2875, 105.5924) ccw
  arc A410 (167.6889, 99.1972) -> (168.1752, 99.2435) centre (167.2136, 106.7696) ccw
  arc A411 (167.383, 100.6616) -> (167.693, 100.6772) centre (167.2735, 105.9324) ccw
  arc A412 (167.693, 100.6772) -> (168.085, 100.7207) centre (167.1831, 107.0646) ccw
  arc A413 (168.085, 100.7207) -> (168.5662, 100.8049) centre (167.017, 108.2324) ccw
  arc A414 (167.6652, 102.1565) -> (167.973, 102.1964) centre (167.1425, 107.4025) ccw
  arc A415 (167.973, 102.1964) -> (168.3604, 102.2705) centre (166.9635, 108.5241) ccw
  arc A416 (168.3604, 102.2705) -> (168.8335, 102.3922) centre (166.7064, 109.6753) ccw
  arc A417 (167.8292, 103.669) -> (168.133, 103.7329) centre (166.8965, 108.8577) ccw
  arc A418 (168.133, 103.7329) -> (168.5133, 103.8371) centre (166.6301, 109.9618) ccw
  arc A419 (168.5133, 103.8371) -> (168.9754, 103.9956) centre (166.2834, 111.0894) ccw
  arc A420 (167.8741, 105.1896) -> (168.1719, 105.2771) centre (166.5371, 110.2892) ccw
  arc A421 (168.1719, 105.2771) -> (168.5429, 105.4109) centre (166.1849, 111.369) ccw
  arc A422 (168.5429, 105.4109) -> (168.9911, 105.6052) centre (165.7508, 112.4658) ccw
  arc A423 (167.7995, 106.7091) -> (168.0895, 106.8197) centre (166.0665, 111.6881) ccw
  arc A424 (168.0895, 106.8197) -> (168.4489, 106.9822) centre (165.6307, 112.7369) ccw
  arc A425 (168.4489, 106.9822) -> (168.8804, 107.2111) centre (165.1119, 113.7963) ccw
  arc A426 (167.6059, 108.2181) -> (167.8863, 108.3511) centre (165.4876, 113.0457) ccw
  arc A427 (167.8863, 108.3511) -> (168.2318, 108.5413) centre (164.9708, 114.0571) ccw
  arc A428 (168.2318, 108.5413) -> (168.6441, 108.8033) centre (164.3705, 115.0726) ccw
  arc A429 (167.2945, 109.7072) -> (167.5636, 109.8618) centre (164.804, 114.3537) ccw
  arc A430 (167.5636, 109.8618) -> (167.8932, 110.0785) centre (164.2095, 115.3215) ccw
  arc A431 (167.8932, 110.0785) -> (168.2836, 110.372) centre (163.5313, 116.2867) ccw
  arc A432 (166.8672, 111.1673) -> (167.1234, 111.3425) centre (164.0199, 115.6041) ccw
  arc A433 (167.1234, 111.3425) -> (167.4349, 111.5844) centre (163.3512, 116.5222) ccw
  arc A434 (167.4349, 111.5844) -> (167.8011, 111.9077) centre (162.5994, 117.4312) ccw
  arc A435 (166.3267, 112.5893) -> (166.5684, 112.7842) centre (163.14, 116.7891) ccw
  arc A436 (166.5684, 112.7842) -> (166.86, 113.0497) centre (162.4014, 117.6519) ccw
  arc A437 (166.86, 113.0497) -> (167.1997, 113.4007) centre (161.5806, 118.4991) ccw
  arc A438 (165.6763, 113.9646) -> (165.9019, 114.1778) centre (162.1699, 117.9014) ccw
  arc A439 (165.9019, 114.1778) -> (166.1718, 114.4654) centre (161.3659, 118.7036) ccw
  arc A440 (166.1718, 114.4654) -> (166.4829, 114.842) centre (160.4812, 119.4838) ccw
  arc A441 (164.92, 115.2846) -> (165.1282, 115.5148) centre (161.1156, 118.9341) ccw
  arc A442 (165.1282, 115.5148) -> (165.3747, 115.8227) centre (160.2511, 119.6708) ccw
  arc A443 (165.3747, 115.8227) -> (165.6553, 116.2226) centre (159.3078, 120.3792) ccw
  arc A444 (164.0625, 116.5412) -> (164.252, 116.7871) centre (159.9834, 119.881) ccw
  arc A445 (164.252, 116.7871) -> (164.4735, 117.1134) centre (159.0638, 120.5476) ccw
  arc A446 (164.4735, 117.1134) -> (164.7219, 117.534) centre (158.0679, 121.1798) ccw
  arc A447 (163.109, 117.7266) -> (163.2786, 117.9866) centre (158.7805, 120.7361) ccw
  arc A448 (163.2786, 117.9866) -> (163.4738, 118.3293) centre (157.8114, 121.3285) ccw
  arc A449 (163.4738, 118.3293) -> (163.6885, 118.7681) centre (156.7689, 121.8806) ccw
  arc A450 (162.0655, 118.8336) -> (162.2141, 119.1061) centre (157.5141, 121.4942) ccw
  arc A451 (162.2141, 119.1061) -> (162.3819, 119.463) centre (156.5015, 122.0087) ccw
  arc A452 (162.3819, 119.463) -> (162.5614, 119.9173) centre (155.419, 122.4773) ccw
  arc A453 (160.9383, 119.8553) -> (161.0651, 120.1386) centre (156.1922, 122.1506) ccw
  arc A454 (161.0651, 120.1386) -> (161.2043, 120.5076) centre (155.1424, 122.5841) ccw
  arc A455 (161.2043, 120.5076) -> (161.3477, 120.9746) centre (154.0264, 122.9663) ccw
  arc A456 (159.7344, 120.7854) -> (159.8386, 121.0778) centre (154.8229, 122.7012) ccw
  arc A457 (159.8386, 121.0778) -> (159.9485, 121.4566) centre (153.7423, 123.051) ccw
  arc A458 (159.9485, 121.4566) -> (160.0547, 121.9334) centre (152.5998, 123.3445) ccw
  arc A459 (158.4612, 121.6182) -> (158.5422, 121.9178) centre (153.4146, 123.1428) ccw
  arc A460 (158.5422, 121.9178) -> (158.622, 122.3041) centre (152.3099, 123.4067) ccw
  arc A461 (158.622, 122.3041) -> (158.6905, 122.7877) centre (151.1478, 123.6096) ccw
  arc A462 (157.1267, 122.3485) -> (157.1839, 122.6536) centre (151.976, 123.4724) ccw
  arc A463 (157.1839, 122.6536) -> (157.2331, 123.0449) centre (150.8539, 123.6488) ccw
  arc A464 (157.2331, 123.0449) -> (157.2635, 123.5324) centre (149.6796, 123.76) ccw
  arc A465 (155.7389, 122.9719) -> (155.772, 123.2805) centre (150.5159, 123.6882) ccw
  arc A466 (155.772, 123.2805) -> (155.7904, 123.6745) centre (149.3835, 123.776) ccw
  arc A467 (155.7904, 123.6745) -> (155.7825, 124.1629) centre (148.2041, 123.7947) ccw
  arc A468 (154.3066, 123.4844) -> (154.3154, 123.7947) centre (149.0434, 123.7888) ccw
  arc A469 (154.3154, 123.7947) -> (154.3028, 124.1889) centre (147.9076, 123.7875) ccw
  arc A470 (154.3028, 124.1889) -> (154.2565, 124.6752) centre (146.7304, 123.7136) ccw
  arc A471 (152.8384, 123.883) -> (152.8228, 124.193) centre (147.5676, 123.7735) ccw
  arc A472 (152.8228, 124.193) -> (152.7793, 124.585) centre (146.4354, 123.6831) ccw
  arc A473 (152.7793, 124.585) -> (152.6951, 125.0662) centre (145.2676, 123.517) ccw
  arc A474 (151.3435, 124.1652) -> (151.3036, 124.473) centre (146.0975, 123.6425) ccw
  arc A475 (151.3036, 124.473) -> (151.2295, 124.8604) centre (144.9759, 123.4635) ccw
  arc A476 (151.2295, 124.8604) -> (151.1078, 125.3335) centre (143.8247, 123.2064) ccw
  arc A477 (149.831, 124.3292) -> (149.7671, 124.633) centre (144.6423, 123.3965) ccw
  arc A478 (149.7671, 124.633) -> (149.6629, 125.0133) centre (143.5382, 123.1301) ccw
  arc A479 (149.6629, 125.0133) -> (149.5044, 125.4754) centre (142.4106, 122.7834) ccw
  arc A480 (148.6896, 124.3741) -> (148.3104, 124.3741) centre (148.5, 105) ccw
  arc A481 (147.169, 124.3292) -> (146.7909, 124.2995) centre (148.5, 105) ccw
  arc A482 (145.6565, 124.1652) -> (145.2819, 124.1059) centre (148.5, 105) ccw
  arc A483 (144.1616, 123.883) -> (143.7928, 123.7945) centre (148.5, 105) ccw
  arc A484 (142.6934, 123.4844) -> (142.3327, 123.3672) centre (148.5, 105) ccw
  arc A485 (141.2611, 122.9719) -> (140.9107, 122.8267) centre (148.5, 105) ccw
  arc A486 (139.8733, 122.3485) -> (139.5354, 122.1763) centre (148.5, 105) ccw
  arc A487 (138.5388, 121.6182) -> (138.2154, 121.42) centre (148.5, 105) ccw
  arc A488 (137.2656, 120.7854) -> (136.9588, 120.5625) centre (148.5, 105) ccw
  arc A489 (136.0617, 119.8553) -> (135.7734, 119.609) centre (148.5, 105) ccw
  arc A490 (134.9345, 118.8336) -> (134.6664, 118.5655) centre (148.5, 105) ccw
  arc A491 (133.891, 117.7266) -> (133.6447, 117.4383) centre (148.5, 105) ccw
  arc A492 (132.9375, 116.5412) -> (132.7146, 116.2344) centre (148.5, 105) ccw
  arc A493 (132.08, 115.2846) -> (131.8818, 114.9612) centre (148.5, 105) ccw
  arc A494 (131.3237, 113.9646) -> (131.1515, 113.6267) centre (148.5, 105) ccw
  arc A495 (130.6733, 112.5893) -> (130.5281, 112.2389) centre (148.5, 105) ccw
  arc A496 (130.1328, 111.1673) -> (130.0156, 110.8066) centre (148.5, 105) ccw
  arc A497 (129.7055, 109.7072) -> (129.617, 109.3384) centre (148.5, 105) ccw
  arc A498 (129.3941, 108.2181) -> (129.3348, 107.8435) centre (148.5, 105) ccw
  arc A499 (129.2005, 106.7091) -> (129.1708, 106.331) centre (148.5, 105) ccw
  arc A500 (129.1259, 105.1896) -> (129.1259, 104.8104) centre (148.5, 105) ccw
  arc A501 (129.1708, 103.669) -> (129.2005, 103.2909) centre (148.5, 105) ccw
  arc A502 (129.3348, 102.1565) -> (129.3941, 101.7819) centre (148.5, 105) ccw
  arc A503 (129.617, 100.6616) -> (129.7055, 100.2928) centre (148.5, 105) ccw
  arc A504 (130.0156, 99.1934) -> (130.1328, 98.8327) centre (148.5, 105) ccw
  arc A505 (130.5281, 97.7611) -> (130.6733, 97.4107) centre (148.5, 105) ccw
  arc A506 (131.1515, 96.3733) -> (131.3237, 96.0354) centre (148.5, 105) ccw
  arc A507 (131.8818, 95.0388) -> (132.08, 94.7154) centre (148.5, 105) ccw
  arc A508 (132.7146, 93.7656) -> (132.9375, 93.4588) centre (148.5, 105) ccw
  arc A509 (133.6447, 92.5617) -> (133.891, 92.2734) centre (148.5, 105) ccw
  arc A510 (134.6664, 91.4345) -> (134.9345, 91.1664) centre (148.5, 105) ccw
  arc A511 (135.7734, 90.391) -> (136.0617, 90.1447) centre (148.5, 105) ccw
  arc A512 (136.9588, 89.4375) -> (137.2656, 89.2146) centre (148.5, 105) ccw
  arc A513 (138.2154, 88.58) -> (138.5388, 88.3818) centre (148.5, 105) ccw
  arc A514 (139.5354, 87.8237) -> (139.8733, 87.6515) centre (148.5, 105) ccw
  arc A515 (140.9107, 87.1733) -> (141.2611, 87.0281) centre (148.5, 105) ccw
  arc A516 (142.3327, 86.6328) -> (142.6934, 86.5156) centre (148.5, 105) ccw
  arc A517 (143.7928, 86.2055) -> (144.1616, 86.117) centre (148.5, 105) ccw
  arc A518 (145.2819, 85.8941) -> (145.6565, 85.8348) centre (148.5, 105) ccw
  arc A519 (146.7909, 85.7005) -> (147.169, 85.6708) centre (148.5, 105) ccw
  arc A520 (148.3104, 85.6259) -> (148.6896, 85.6259) centre (148.5, 105) ccw
  arc A521 (149.831, 85.6708) -> (150.2091, 85.7005) centre (148.5, 105) ccw
  arc A522 (151.3435, 85.8348) -> (151.7181, 85.8941) centre (148.5, 105) ccw
  arc A523 (152.8384, 86.117) -> (153.2072, 86.2055) centre (148.5, 105) ccw
  arc A524 (154.3066, 86.5156) -> (154.6673, 86.6328) centre (148.5, 105) ccw
  arc A525 (155.7389, 87.0281) -> (156.0893, 87.1733) centre (148.5, 105) ccw
  arc A526 (157.1267, 87.6515) -> (157.4646, 87.8237) centre (148.5, 105) ccw
  arc A527 (158.4612, 88.3818) -> (158.7846, 88.58) centre (148.5, 105) ccw
  arc A528 (159.7344, 89.2146) -> (160.0412, 89.4375) centre (148.5, 105) ccw
  arc A529 (160.9383, 90.1447) -> (161.2266, 90.391) centre (148.5, 105) ccw
  arc A530 (162.0655, 91.1664) -> (162.3336, 91.4345) centre (148.5, 105) ccw
  arc A531 (163.109, 92.2734) -> (163.3553, 92.5617) centre (148.5, 105) ccw
  arc A532 (164.0625, 93.4588) -> (164.2854, 93.7656) centre (148.5, 105) ccw
  arc A533 (164.92, 94.7154) -> (165.1182, 95.0388) centre (148.5, 105) ccw
  arc A534 (165.6763, 96.0354) -> (165.8485, 96.3733) centre (148.5, 105) ccw
  arc A535 (166.3267, 97.4107) -> (166.4719, 97.7611) centre (148.5, 105) ccw
  arc A536 (166.8672, 98.8327) -> (166.9844, 99.1934) centre (148.5, 105) ccw
  arc A537 (167.2945, 100.2928) -> (167.383, 100.6616) centre (148.5, 105) ccw
  arc A538 (167.6059, 101.7819) -> (167.6652, 102.1565) centre (148.5, 105) ccw
  arc A539 (167.7995, 103.2909) -> (167.8292, 103.669) centre (148.5, 105) ccw
  arc A540 (167.8741, 104.8104) -> (167.8741, 105.1896) centre (148.5, 105) ccw
  arc A541 (167.8292, 106.331) -> (167.7995, 106.7091) centre (148.5, 105) ccw
  arc A542 (167.6652, 107.8435) -> (167.6059, 108.2181) centre (148.5, 105) ccw
  arc A543 (167.383, 109.3384) -> (167.2945, 109.7072) centre (148.5, 105) ccw
  arc A544 (166.9844, 110.8066) -> (166.8672, 111.1673) centre (148.5, 105) ccw
  arc A545 (166.4719, 112.2389) -> (166.3267, 112.5893) centre (148.5, 105) ccw
  arc A546 (165.8485, 113.6267) -> (165.6763, 113.9646) centre (148.5, 105) ccw
  arc A547 (165.1182, 114.9612) -> (164.92, 115.2846) centre (148.5, 105) ccw
  arc A548 (164.2854, 116.2344) -> (164.0625, 116.5412) centre (148.5, 105) ccw
  arc A549 (163.3553, 117.4383) -> (163.109, 117.7266) centre (148.5, 105) ccw
  arc A550 (162.3336, 118.5655) -> (162.0655, 118.8336) centre (148.5, 105) ccw
  arc A551 (161.2266, 119.609) -> (160.9383, 119.8553) centre (148.5, 105) ccw
  arc A552 (160.0412, 120.5625) -> (159.7344, 120.7854) centre (148.5, 105) ccw
  arc A553 (158.7846, 121.42) -> (158.4612, 121.6182) centre (148.5, 105) ccw
  arc A554 (157.4646, 122.1763) -> (157.1267, 122.3485) centre (148.5, 105) ccw
  arc A555 (156.0893, 122.8267) -> (155.7389, 122.9719) centre (148.5, 105) ccw
  arc A556 (154.6673, 123.3672) -> (154.3066, 123.4844) centre (148.5, 105) ccw
  arc A557 (153.2072, 123.7945) -> (152.8384, 123.883) centre (148.5, 105) ccw
  arc A558 (151.7181, 124.1059) -> (151.3435, 124.1652) centre (148.5, 105) ccw
  arc A559 (150.2091, 124.2995) -> (149.831, 124.3292) centre (148.5, 105) ccw
  arc A560 (147.8948, 125.4911) -> (147.4956, 125.4754) centre (148.5, 105) ccw
  arc A561 (146.2889, 125.3804) -> (145.8922, 125.3335) centre (148.5, 105) ccw
  arc A562 (144.6967, 125.1441) -> (144.3049, 125.0662) centre (148.5, 105) ccw
  arc A563 (143.128, 124.7836) -> (142.7435, 124.6752) centre (148.5, 105) ccw
  arc A564 (141.5923, 124.3011) -> (141.2175, 124.1629) centre (148.5, 105) ccw
  arc A565 (140.0993, 123.6997) -> (139.7365, 123.5324) centre (148.5, 105) ccw
  arc A566 (138.658, 122.9829) -> (138.3095, 122.7877) centre (148.5, 105) ccw
  arc A567 (137.2774, 122.1553) -> (136.9453, 121.9334) centre (148.5, 105) ccw
  arc A568 (135.966, 121.2219) -> (135.6523, 120.9746) centre (148.5, 105) ccw
  arc A569 (134.7319, 120.1885) -> (134.4386, 119.9173) centre (148.5, 105) ccw
  arc A570 (133.5827, 119.0614) -> (133.3115, 118.7681) centre (148.5, 105) ccw
  arc A571 (132.5254, 117.8477) -> (132.2781, 117.534) centre (148.5, 105) ccw
  arc A572 (131.5666, 116.5547) -> (131.3447, 116.2226) centre (148.5, 105) ccw
  arc A573 (130.7123, 115.1905) -> (130.5171, 114.842) centre (148.5, 105) ccw
  arc A574 (129.9676, 113.7635) -> (129.8003, 113.4007) centre (148.5, 105) ccw
  arc A575 (129.3371, 112.2825) -> (129.1989, 111.9077) centre (148.5, 105) ccw
  arc A576 (128.8248, 110.7565) -> (128.7164, 110.372) centre (148.5, 105) ccw
  arc A577 (128.4338, 109.1951) -> (128.3559, 108.8033) centre (148.5, 105) ccw
  arc A578 (128.1665, 107.6078) -> (128.1196, 107.2111) centre (148.5, 105) ccw
  arc A579 (128.0246, 106.0044) -> (128.0089, 105.6052) centre (148.5, 105) ccw
  arc A580 (128.0089, 104.3948) -> (128.0246, 103.9956) centre (148.5, 105) ccw
  arc A581 (128.1196, 102.7889) -> (128.1665, 102.3922) centre (148.5, 105) ccw